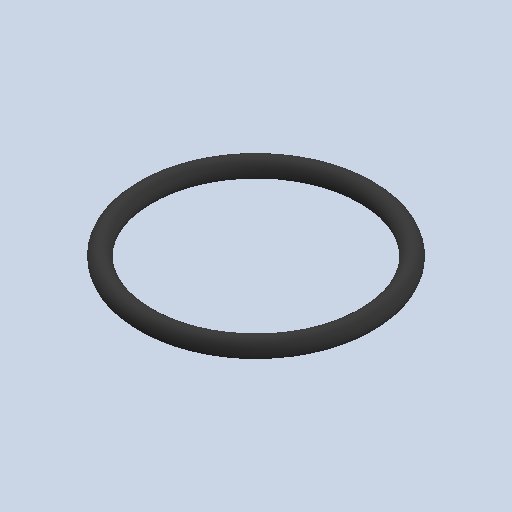
# Autodesk Inventor part: oring
Saved by Autodesk Inventor 2024 (Build 280153000, 153)
## iProperties
Created: 2023-11-04
Part Number: oring
Material: Rubber
Document SubType Name: Modeling
Designer: schanen
Density: 0.93 g/cm^3
Appearance: Rubber - Black
oring_dia: 4.000 mm
Author: schanen
Autodesk Inventor part; units mm, degrees
ref_plane "YZ Plane" through (0, 0, 0) normal (1, 0, 0) x (0, 1, 0)
ref_plane "XZ Plane" through (0, 0, 0) normal (0, 1, 0) x (-1, 0, 0)
ref_plane "XY Plane" through (0, 0, 0) normal (0, 0, 1) x (1, 0, 0)
sketch "Sketch1" plane through (0, 0, 0) normal (0, 0, 1) x (1, 0, 0)
  circle A0 centre (-24.225, 0) radius 2
  line L0 (0, -2.8) -> (0, 2.8) projected
  point P0 (0, 0)
  dimension "oring_dia" = 4
  dimension "d1" = 24.225
  constraints: 1 centre point
  measures "oring_dia" diameter of A0
  measures "d1" distance from line of L0 A0.centre
revolve "Revolution1" add sketch "Sketch1" angle 360 about axis through (0, -10, 0) along (0, 1, 0)
equation "\"d1\" = 0.5 * cylinder_od + 0.5 * oring_dia"
equation "\"cylinder_od\" = 44.45"
body "Solid1"
